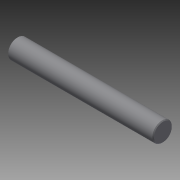
# Autodesk Inventor part: SSS1-10
Saved by Autodesk Inventor 2014 SP2 (Build 180246200, 246)
## iProperties
Created: 2019-04-14
Part Number: SSS1-10
Material: Generic
Catalog Web Link: www.cadenas.de
Description: Spur Pinion Shafts (SSS)-
Vendor: KHK
Document SubType Name: Modeling
Designer: psadmin
Manufacturer: KHK
Mass: 10.1696 g
Surface Area: 35.9638 cm^2
Volume: 10.1696 cm^3
Density: 1 g/cm^3
Appearance: PSOLRGB-175-175-175
Category: PARTsolutions
Company: KHK
Title: SSS1-10
Author: Cadenas PARTsolutions
PSOL_IDENT_0: {$CADENAS_DATA\23d-libs\khk\spur_gears\spur_pinion_shafts_sss.prj},175 {VTYP=3D},{NB=SSS1-10},{LINA=
PSOL_IDENT_1: SSS1-10},{NN=Spur Pinion Shafts (SSS)},{DATE=15.02.2019 02:43:12},{GEOMDATE=28.11.2008 13:19:00},{VE
PSOL_IDENT_2: RSION=},{LINEID=15070},{WBVAR=},{WBNUMERIC=}  {NB=SSS1-10},{LINA=SSS1-10},{KT=DUMMY},{CN=SSS1-10},{M=
PSOL_IDENT_3: 1.0},{Z=10},{TC=0.0},{F2=0},{A2=0.0},{C=10.0},{D=12.0},{E=12},{A=12.0},{F=78},{G=90},{S=SA},{X=1}
NN: Spur Pinion Shafts (SSS)
NB: SSS1-10
NBSYN: $CN.
LINA: SSS1-10
CN: SSS1-10
M: 1
Z: 10
TC: 0
F2: 0
A2: 0
C: 10
D: 12
E: 12
A: 12
F: 78
G: 90
S: SA
SUPPLIER: KHK
ARTICLENO: SSS1-10
BOMINFO: SSS1-10
CREATOR: CADENAS GmbH
Autodesk Inventor part; units mm, degrees
ref_plane "YZ Plane" through (0, 0, 0) normal (1, 0, 0) x (0, 1, 0)
ref_plane "XZ Plane" through (0, 0, 0) normal (0, 1, 0) x (-1, 0, 0)
ref_plane "XY Plane" through (0, 0, 0) normal (0, 0, 1) x (1, 0, 0)
sketch "Sketch_1" plane through (0, 0, 0) normal (0, 0, 1) x (1, 0, 0)
  line L0 (90, 0) -> (0, 0)
  line L1 (0, 0) -> (0, 5.5)
  line L2 (0, 5.5) -> (0.5, 6)
  line L3 (0.5, 6) -> (89.5, 6)
  line L4 (89.5, 6) -> (90, 5.5)
  line L5 (90, 5.5) -> (90, 0)
  line L6 (90, 0) -> (0, 0)
  constraints: 14 end point
revolve "Revolution1" add sketch "Sketch_1" angle 360 about axis through (90, 0, 0) along (1, 0, 0)
body "Solid1"
